Autodesk Inventor part; units mm, degrees
(part 2 of 2)
  line L135 (29.2243, -208.6026) -> (30.7211, -208.6026)
  line L136 (30.7211, -208.6026) -> (30.7211, -208.9558)
  spline S178 degree 2 poles (33.0256, -207.4318) (33.0256, -208.2519) (32.5489, -209.02) (32.0524, -209.02) knots 0 0 0 1 2 2 2
  spline S179 degree 2 poles (32.0524, -209.02) (31.5486, -209.02) (31.0768, -208.237) (31.0768, -207.4343) knots 0 0 0 1 2 2 2
  spline S180 degree 2 poles (31.0768, -207.4343) (31.0768, -206.6093) (31.5535, -205.8461) (32.0524, -205.8461) knots 0 0 0 1 2 2 2
  spline S181 degree 2 poles (32.0524, -205.8461) (32.5539, -205.8461) (33.0256, -206.6365) (33.0256, -207.4318) knots 0 0 0 1 2 2 2
  spline S182 degree 2 poles (32.502, -208.3605) (32.5613, -208.2099) (32.6107, -207.7455) (32.6107, -207.4318) knots 0 0 0 1 2 2 2
  spline S183 degree 2 poles (32.6107, -207.4318) (32.6107, -207.1181) (32.5613, -206.6562) (32.4995, -206.5006) knots 0 0 0 1 2 2 2
  spline S184 degree 2 poles (32.4995, -206.5006) (32.4378, -206.345) (32.2229, -206.1845) (32.0524, -206.1845) knots 0 0 0 1 2 2 2
  spline S185 degree 2 poles (32.0524, -206.1845) (31.882, -206.1845) (31.6622, -206.345) (31.598, -206.5056) knots 0 0 0 1 2 2 2
  spline S186 degree 2 poles (31.598, -206.5056) (31.5362, -206.6612) (31.4917, -207.1354) (31.4917, -207.4343) knots 0 0 0 1 2 2 2
  spline S187 degree 2 poles (31.4917, -207.4343) (31.4917, -207.7554) (31.5313, -208.1852) (31.5955, -208.3531) knots 0 0 0 1 2 2 2
  spline S188 degree 2 poles (31.5955, -208.3531) (31.6548, -208.5112) (31.8746, -208.6816) (32.0524, -208.6816) knots 0 0 0 1 2 2 2
  spline S189 degree 2 poles (32.0524, -208.6816) (32.2204, -208.6816) (32.4402, -208.5211) (32.502, -208.3605) knots 0 0 0 1 2 2 2
  line L137 (35.2956, -208.9558) -> (33.4159, -208.9558)
  line L138 (33.4159, -208.9558) -> (33.4159, -208.5236)
  spline S190 degree 2 poles (33.4159, -208.5236) (33.6184, -208.3334) (33.9791, -207.9802) (34.152, -207.79) knots 0 0 0 1 2 2 2
  spline S191 degree 2 poles (34.152, -207.79) (34.5002, -207.4071) (34.7546, -206.9477) (34.7546, -206.7032) knots 0 0 0 1 2 2 2
  spline S192 degree 2 poles (34.7546, -206.7032) (34.7546, -206.5747) (34.6756, -206.3821) (34.604, -206.3203) knots 0 0 0 1 2 2 2
  spline S193 degree 2 poles (34.604, -206.3203) (34.5323, -206.2586) (34.3446, -206.1968) (34.231, -206.1968) knots 0 0 0 1 2 2 2
  spline S194 degree 2 poles (34.231, -206.1968) (34.1223, -206.1968) (33.9, -206.2512) (33.7987, -206.2931) knots 0 0 0 1 2 2 2
  spline S195 degree 2 poles (33.7987, -206.2931) (33.7123, -206.3277) (33.5517, -206.4265) (33.5023, -206.4611) knots 0 0 0 1 2 2 2
  line L139 (33.5023, -206.4611) -> (33.4801, -206.4611)
  line L140 (33.4801, -206.4611) -> (33.4801, -206.0264)
  spline S196 degree 2 poles (33.4801, -206.0264) (33.6061, -205.9646) (34.0581, -205.8436) (34.2606, -205.8436) knots 0 0 0 1 2 2 2
  spline S197 degree 2 poles (34.2606, -205.8436) (34.6879, -205.8436) (35.1696, -206.2956) (35.1696, -206.6809) knots 0 0 0 1 2 2 2
  spline S198 degree 2 poles (35.1696, -206.6809) (35.1696, -206.8612) (35.0856, -207.1626) (35.0115, -207.291) knots 0 0 0 1 2 2 2
  spline S199 degree 2 poles (35.0115, -207.291) (34.9374, -207.4244) (34.7225, -207.6862) (34.604, -207.8122) knots 0 0 0 1 2 2 2
  spline S200 degree 2 poles (34.604, -207.8122) (34.4113, -208.0222) (33.9395, -208.4717) (33.7987, -208.6026) knots 0 0 0 1 2 2 2
  line L141 (33.7987, -208.6026) -> (35.2956, -208.6026)
  line L142 (35.2956, -208.6026) -> (35.2956, -208.9558)
  spline S201 degree 2 poles (37.6297, -207.9678) (37.6297, -208.2025) (37.4741, -208.6001) (37.3432, -208.7335) knots 0 0 0 1 2 2 2
  spline S202 degree 2 poles (37.3432, -208.7335) (37.2074, -208.8743) (36.8665, -209.02) (36.6615, -209.02) knots 0 0 0 1 2 2 2
  spline S203 degree 2 poles (36.6615, -209.02) (36.4565, -209.02) (36.1181, -208.8817) (35.9896, -208.7434) knots 0 0 0 1 2 2 2
  spline S204 degree 2 poles (35.9896, -208.7434) (35.8316, -208.5779) (35.6537, -208.0222) (35.6537, -207.6171) knots 0 0 0 1 2 2 2
  spline S205 degree 2 poles (35.6537, -207.6171) (35.6537, -207.2194) (35.8167, -206.5797) (35.9872, -206.3425) knots 0 0 0 1 2 2 2
  spline S206 degree 2 poles (35.9872, -206.3425) (36.1527, -206.1104) (36.6763, -205.851) (37.0196, -205.851) knots 0 0 0 1 2 2 2
  spline S207 degree 2 poles (37.0196, -205.851) (37.1209, -205.851) (37.2988, -205.8708) (37.3654, -205.893) knots 0 0 0 1 2 2 2
  line L143 (37.3654, -205.893) -> (37.3654, -206.2857)
  line L144 (37.3654, -206.2857) -> (37.3482, -206.2857)
  spline S208 degree 2 poles (37.3482, -206.2857) (37.2913, -206.2561) (37.0839, -206.2042) (36.9653, -206.2042) knots 0 0 0 1 2 2 2
  spline S209 degree 2 poles (36.9653, -206.2042) (36.5849, -206.2042) (36.1181, -206.718) (36.0736, -207.2219) knots 0 0 0 1 2 2 2
  spline S210 degree 2 poles (36.0736, -207.2219) (36.2194, -207.1206) (36.5256, -207.0094) (36.7084, -207.0094) knots 0 0 0 1 2 2 2
  spline S211 degree 2 poles (36.7084, -207.0094) (36.8863, -207.0094) (37.153, -207.0811) (37.2988, -207.1898) knots 0 0 0 1 2 2 2
  spline S212 degree 2 poles (37.2988, -207.1898) (37.4667, -207.3157) (37.6297, -207.706) (37.6297, -207.9678) knots 0 0 0 1 2 2 2
  spline S213 degree 2 poles (37.2148, -207.9851) (37.2148, -207.7974) (37.116, -207.543) (37.0073, -207.454) knots 0 0 0 1 2 2 2
  spline S214 degree 2 poles (37.0073, -207.454) (36.9258, -207.3898) (36.7232, -207.3478) (36.617, -207.3478) knots 0 0 0 1 2 2 2
  spline S215 degree 2 poles (36.617, -207.3478) (36.4738, -207.3478) (36.2045, -207.4343) (36.0736, -207.5158) knots 0 0 0 1 2 2 2
  spline S216 degree 2 poles (36.0736, -207.5158) (36.0712, -207.5603) (36.0662, -207.6442) (36.0662, -207.7085) knots 0 0 0 1 2 2 2
  spline S217 degree 2 poles (36.0662, -207.7085) (36.0662, -208.0246) (36.1897, -208.4124) (36.2836, -208.5137) knots 0 0 0 1 2 2 2
  spline S218 degree 2 poles (36.2836, -208.5137) (36.37, -208.61) (36.5578, -208.6866) (36.664, -208.6866) knots 0 0 0 1 2 2 2
  spline S219 degree 2 poles (36.664, -208.6866) (36.911, -208.6866) (37.2148, -208.3358) (37.2148, -207.9851) knots 0 0 0 1 2 2 2
  point P0 (0, 0)
  constraints: 2 other
emboss "Emboss1" sketch "Sketch14" operation cut depth 2.54 direction (-1, 0, 0)
sketch "Sketch16" plane through (5.08, 0, 0) normal (1, 0, 0) x (0, 0, -1)
  line L0 (-41.7074, -74.9522) -> (39.5726, -74.9522)
  line L1 (39.5726, -74.9522) -> (39.5726, -78.7622)
  line L2 (39.5726, -78.7622) -> (-41.7074, -78.7622)
  line L3 (-41.7074, -78.7622) -> (-41.7074, -74.9522)
  line L4 (22.7938, -210.0802) -> (-43.6417, -210.0802) projected
  point P0 (0, 0)
  point P1 (-43.6417, -212.6202)
  dimension "d193" = 135.128
  dimension "d195" = 3.81
  constraints: 8 end point, 2 parallel, 1 horizontal, 1 perpendicular
  measures "d193" distance between parallel lines of L4 L0
  measures "d195" distance between parallel lines of L0 L2
extrude "Extrusion13" add sketch "Sketch16" along normal blind 5.08
sketch "Sketch17" plane through (22.86, 33.2264, 20.9087) normal (0, 1, 0) x (1, 0, 0)
  line L0 (-6.858, 35.56) -> (0, 35.56) projected
  line L1 (-0.0061, 35.56) -> (0.0392, 35.56)
  line L2 (0, 64.9986) -> (0, -27.9146) projected
  line L3 (0, 35.5801) -> (0, 35.5243)
  line L4 (5, -24.7396) -> (5, 61.8236) projected
  line L5 (0, 35.56) -> (5, 35.56)
  line L6 (5, 35.56) -> (5, -0.0031)
  line L7 (5, -0.0031) -> (0, -0.0031)
  line L8 (0, -0.0031) -> (0, 35.56)
  point P0 (-22.86, 20.9087)
  point P1 (5, -23.8506)
  point P2 (5, 69.0626)
  point P3 (0.0392, 35.56)
  constraints: 12 end point, 4 point on line, 2 horizontal, 2 parallel, 1 perpendicular
extrude "Extrusion14" cut sketch "Sketch17" against normal blind 2.0066
sketch "Sketch18" plane through (0, 0, 0) normal (-1, 0, 0) x (0, 0, 1)
  arc A0 (46.2144, 33.1755) -> (48.7724, 30.6175) centre (48.0867, 32.4898) ccw projected
  circle A1 centre (48.0867, 32.4898) radius 4.5085
  arc A2 (-41.481, 33.1755) -> (-44.039, 30.6175) centre (-43.3533, 32.4898) ccw projected
  circle A3 centre (-43.3533, 32.4898) radius 4.5085
  arc A4 (-44.039, -212.018) -> (-41.481, -214.576) centre (-43.3533, -213.8902) ccw projected
  circle A5 centre (-43.3533, -213.8902) radius 4.5085
  arc A6 (46.2144, -214.576) -> (48.7724, -212.018) centre (48.0867, -213.8902) ccw projected
  circle A7 centre (48.0867, -213.8902) radius 4.5085
  point P0 (0, 0)
  dimension "d209" = 9.017
  dimension "d210" = 9.017
  dimension "d211" = 9.017
  dimension "d212" = 9.017
  constraints: 4 centre point, 4 coincident
  measures "d209" diameter of A1
  measures "d210" diameter of A3
  measures "d211" diameter of A5
  measures "d212" diameter of A7
extrude "Extrusion15" [suppressed]
sketch "Sketch19" plane through (22.86, -68.6784, -44.0899) normal (0, 0, -1) x (-1, 0, 0)
  line L0 (6.35, 0) -> (0, 0) projected
  line L1 (-5, 96.7232) -> (-5, -140.7668) projected
  line L2 (0, 0) -> (-5, 0)
  line L3 (-5, 0) -> (-5, 8.001)
  line L4 (-5, 8.001) -> (0, 8.001)
  line L5 (0, 8.001) -> (0, 0)
  point P0 (22.86, 68.6784)
  dimension "d216" = 5
  dimension "d219" = 8.001
  constraints: 8 end point, 2 parallel, 1 horizontal, 1 perpendicular, 1 point on line
  measures "d216" distance between parallel lines of L1 L5
  measures "d219" distance between parallel lines of L2 L4
extrude "Extrusion16" cut sketch "Sketch19" against normal blind 24.13
sketch "Sketch20" plane through (0, 0, 0) normal (-1, 0, 0) x (0, 0, 1)
  line L0 (-45.1249, 28.9592) -> (-41.5943, 28.9592)
  line L1 (-45.1249, 36.0204) -> (-41.5943, 36.0204)
  line L2 (-45.1249, 28.9592) -> (-47.1633, 32.4898)
  line L3 (-45.1249, 36.0204) -> (-47.1633, 32.4898)
  line L4 (-41.5943, 28.9592) -> (-39.5559, 32.4898)
  line L5 (-41.5943, 36.0204) -> (-39.5559, 32.4898)
  line L6 (49.8457, 36.0204) -> (51.8841, 32.4898)
  line L7 (49.8457, 28.9592) -> (51.8841, 32.4898)
  line L8 (46.3151, 28.9592) -> (49.8457, 28.9592)
  line L9 (46.3151, 36.0204) -> (49.8457, 36.0204)
  line L10 (46.3151, 36.0204) -> (44.2767, 32.4898)
  line L11 (46.3151, 28.9592) -> (44.2767, 32.4898)
  line L12 (-41.5943, -210.3596) -> (-39.5559, -213.8902)
  line L13 (-41.5943, -217.4208) -> (-39.5559, -213.8902)
  line L14 (-45.1249, -217.4208) -> (-41.5943, -217.4208)
  line L15 (-45.1249, -210.3596) -> (-41.5943, -210.3596)
  line L16 (-45.1249, -210.3596) -> (-47.1633, -213.8902)
  line L17 (-45.1249, -217.4208) -> (-47.1633, -213.8902)
  line L18 (49.8457, -210.3596) -> (51.8841, -213.8902)
  line L19 (49.8457, -217.4208) -> (51.8841, -213.8902)
  line L20 (46.3151, -217.4208) -> (49.8457, -217.4208)
  line L21 (46.3151, -210.3596) -> (49.8457, -210.3596)
  line L22 (46.3151, -210.3596) -> (44.2767, -213.8902)
  line L23 (46.3151, -217.4208) -> (44.2767, -213.8902)
  line L24 (-40.0449, -45.2596) -> (-36.5143, -45.2596)
  line L25 (-36.5143, -45.2596) -> (-34.4759, -48.7902)
  line L26 (-40.0449, -45.2596) -> (-42.0833, -48.7902)
  line L27 (-36.5143, -52.3208) -> (-34.4759, -48.7902)
  line L28 (-40.0449, -52.3208) -> (-42.0833, -48.7902)
  line L29 (-40.0449, -52.3208) -> (-36.5143, -52.3208)
  line L30 (41.2351, -45.2596) -> (39.1967, -48.7902)
  line L31 (41.2351, -52.3208) -> (39.1967, -48.7902)
  line L32 (41.2351, -45.2596) -> (44.7657, -45.2596)
  line L33 (41.2351, -52.3208) -> (44.7657, -52.3208)
  line L34 (44.7657, -52.3208) -> (46.8041, -48.7902)
  line L35 (44.7657, -45.2596) -> (46.8041, -48.7902)
  point P0 (0, 0)
  point P1 (-43.3596, 28.9592)
  point P2 (-43.3533, 32.4898)
  point P3 (48.0804, 28.9592)
  point P4 (-43.3596, -217.4208)
  point P5 (48.0804, -217.4208)
  point P6 (-38.2796, -52.3208)
  point P7 (-38.2733, -48.7902)
  point P8 (43.0004, -52.3208)
  point P9 (43.0067, -48.7902)
  dimension "d366" = 7.0612
  dimension "d367" = 120
  dimension "d368" = 120
  dimension "d369" = 120
  dimension "d370" = 120
  dimension "d371" = 3.5306
  dimension "d372" = 3.5306
  dimension "d373" = 3.5306
  dimension "d374" = 3.5306
  dimension "d375" = 3.5306
  dimension "d376" = 3.5306
  dimension "d377" = 0
  dimension "d378" = 7.6074
  dimension "d383" = 7.0612
  dimension "d384" = 120
  dimension "d385" = 120
  dimension "d386" = 120
  dimension "d387" = 120
  dimension "d388" = 3.5306
  dimension "d389" = 3.5306
  dimension "d390" = 3.5306
  dimension "d391" = 3.5306
  dimension "d392" = 3.5306
  dimension "d393" = 3.5306
  dimension "d394" = 0
  dimension "d395" = 7.6074
  dimension "d402" = 7.0612
  dimension "d403" = 120
  dimension "d404" = 120
  dimension "d405" = 120
  dimension "d406" = 120
  dimension "d407" = 3.5306
  dimension "d408" = 3.5306
  dimension "d409" = 3.5306
  dimension "d410" = 3.5306
  dimension "d411" = 3.5306
  dimension "d412" = 3.5306
  dimension "d413" = 0
  dimension "d414" = 7.6074
  dimension "d421" = 7.0612
  dimension "d422" = 120
  dimension "d423" = 120
  dimension "d424" = 120
  dimension "d425" = 120
  dimension "d426" = 3.5306
  dimension "d427" = 3.5306
  dimension "d428" = 3.5306
  dimension "d429" = 3.5306
  dimension "d430" = 3.5306
  dimension "d431" = 3.5306
  dimension "d432" = 0
  dimension "d433" = 7.6074
  dimension "d629" = 7.0612
  dimension "d630" = 120
  dimension "d631" = 120
  dimension "d632" = 120
  dimension "d633" = 120
  dimension "d634" = 3.5306
  dimension "d635" = 3.5306
  dimension "d636" = 3.5306
  dimension "d637" = 3.5306
  dimension "d638" = 3.5306
  dimension "d639" = 3.5306
  dimension "d640" = 0
  constraints: 72 end point, 12 horizontal, 6 midpoint
  measures "d366" distance from line of point (-43.36, 28.959) L1
  measures "d367" angle of L0 L2
  measures "d368" angle of L1 L3
  measures "d369" angle of L4 L0
  measures "d370" angle of L5 L1
  measures "d371" distance of L0.start L4.start
  measures "d372" distance of L1.start L5.start
  measures "d373" vertical distance of L1.start L3.end
  measures "d374" vertical distance of L0.start L2.end
  measures "d375" vertical distance of L5.start L5.end
  measures "d376" vertical distance of L4.start L4.end
  measures "d377" horizontal distance of L0.start L1.start
  measures "d378" distance of L4.end L2.end
  measures "d383" distance from line of point (48.08, 28.959) L9
  measures "d384" angle of L8 L11
  measures "d385" angle of L9 L10
  measures "d386" angle of L7 L8
  measures "d387" angle of L6 L9
  measures "d388" distance of L8.start L7.start
  measures "d389" distance of L9.start L6.start
  measures "d390" vertical distance of L9.start L10.end
  measures "d391" vertical distance of L8.start L11.end
  measures "d392" vertical distance of L6.start L6.end
  measures "d393" vertical distance of L7.start L7.end
  measures "d394" horizontal distance of L8.start L9.start
  measures "d395" distance of L7.end L11.end
  measures "d402" distance from line of point (-43.36, -217.421) L15
  measures "d403" angle of L14 L17
  measures "d404" angle of L15 L16
  measures "d405" angle of L13 L14
  measures "d406" angle of L12 L15
  measures "d407" distance of L14.start L13.start
  measures "d408" distance of L15.start L12.start
  measures "d409" vertical distance of L15.start L16.end
  measures "d410" vertical distance of L14.start L17.end
  measures "d411" vertical distance of L12.start L12.end
  measures "d412" vertical distance of L13.start L13.end
  measures "d413" horizontal distance of L14.start L15.start
  measures "d414" distance of L13.end L17.end
  measures "d421" distance from line of point (48.08, -217.421) L21
  measures "d422" angle of L20 L23
  measures "d423" angle of L21 L22
  measures "d424" angle of L19 L20
  measures "d425" angle of L18 L21
  measures "d426" distance of L20.start L19.start
  measures "d427" distance of L21.start L18.start
  measures "d428" vertical distance of L21.start L22.end
  measures "d429" vertical distance of L20.start L23.end
  measures "d430" vertical distance of L18.start L18.end
  measures "d431" vertical distance of L19.start L19.end
  measures "d432" horizontal distance of L20.start L21.start
  measures "d433" distance of L19.end L23.end
  measures "d629" distance from line of point (-38.28, -52.321) L24
  measures "d630" angle of L29 L28
  measures "d631" angle of L24 L26
  measures "d632" angle of L27 L29
  measures "d633" angle of L25 L24
  measures "d634" distance of L28.start L29.end
  measures "d635" distance of L26.start L24.end
  measures "d636" vertical distance of L26.start L26.end
  measures "d637" vertical distance of L28.start L28.end
  measures "d638" vertical distance of L24.end L25.end
  measures "d639" vertical distance of L29.end L27.end
  measures "d640" horizontal distance of L28.start L26.start
extrude "Extrusion18" cut sketch "Sketch20" against normal blind 4
sketch "Sketch21" plane through (5.08, 0, 0) normal (1, 0, 0) x (0, 0, -1)
  line L0 (42.0833, 28.0448) -> (42.0833, -209.4452) projected
  line L1 (-46.2035, -59.6599) -> (-46.8167, -60.8152)
  line L2 (-41.6901, -56.7111) -> (-44.8426, -58.3204)
  arc A0 (-44.8426, -58.3204) -> (-46.2035, -59.6599) centre (-43.399, -61.1483) ccw
  line L3 (-46.2187, -55.0206) -> (-46.361, -55.3921)
  arc A1 (-41.6901, -56.7111) -> (-39.9587, -53.8833) centre (-43.1337, -53.8833) ccw
  line L4 (-39.9587, -43.7605) -> (-39.9587, -53.8833)
  arc A2 (-39.9587, -43.7605) -> (-41.6901, -40.9327) centre (-43.1337, -43.7605) ccw
  line L5 (-41.6901, -40.9327) -> (-44.8426, -39.3233)
  line L6 (-46.2035, -37.9839) -> (-46.8167, -36.8286)
  arc A3 (-46.2035, -37.9839) -> (-44.8426, -39.3233) centre (-43.399, -36.4955) ccw
  line L7 (-46.8167, -209.4452) -> (-46.8167, 28.0448) projected
  line L8 (-46.8167, -36.8286) -> (-46.8167, -60.8152)
  circle A4 centre (-43.0067, -48.7902) radius 1.9939
  line L9 (35.2253, -54.5067) -> (35.2253, -44.384)
  line L10 (42.0833, -37.452) -> (42.0833, -61.4386)
  circle A5 centre (38.2733, -48.7902) radius 1.9939
  line L11 (42.0833, -41.6782) -> (42.0833, -55.9022)
  line L12 (35.2282, -53.9583) -> (35.2282, -43.6222)
  line L13 (36.9596, -40.7944) -> (40.1092, -39.1865)
  line L14 (41.4701, -37.8471) -> (42.0833, -36.6918)
  line L15 (36.9596, -56.7861) -> (40.1092, -58.394)
  line L16 (41.4701, -59.7334) -> (42.0833, -60.8887)
  arc A6 (36.9596, -40.7944) -> (35.2282, -43.6222) centre (38.4032, -43.6222) ccw
  arc A7 (40.1092, -39.1865) -> (41.4701, -37.8471) centre (38.6656, -36.3587) ccw
  arc A8 (35.2282, -53.9583) -> (36.9596, -56.7861) centre (38.4032, -53.9583) ccw
  arc A9 (41.4701, -59.7334) -> (40.1092, -58.394) centre (38.6656, -61.2218) ccw
  point P0 (0, 0)
  point P1 (-45.7342, -58.7756)
  point P2 (-43.0182, -55.9022)
  point P3 (-45.7342, -38.8682)
  point P4 (-43.0182, -41.6782)
  point P5 (41.0008, -38.7314)
  point P6 (41.0008, -58.8491)
  dimension "d568" = 14.224
  dimension "d569" = 2.0396
  dimension "d570" = 2.0396
  dimension "d571" = 145
  dimension "d572" = 145
  dimension "d574" = 117.044
  dimension "d575" = 117.044
  dimension "d576" = 3.175
  dimension "d577" = 6.858
  dimension "d578" = 6.858
  dimension "d579" = 7.112
  dimension "d593" = 6.858
  dimension "d594" = 6.858
  dimension "d595" = 3.9878
  dimension "d596" = 3.9878
  dimension "d598" = 0
  dimension "d600" = 3.1525
  dimension "d601" = 2.0396
  dimension "d602" = 2.0396
  dimension "d603" = 117.044
  dimension "d604" = 117.044
  dimension "d606" = 3.175
  dimension "d607" = 3.1496
  dimension "d608" = 3.1496
  dimension "d609" = 145
  dimension "d611" = 145
  constraints: 30 end point, 16 point on circle, 16 tangent, 10 centre point, 9 point on line, 6 equal radius, 2 coincident, 2 vertical, 1 parallel
  measures "d568" distance of point (-43.018, -55.902) point (-43.018, -41.678)
  measures "d569" vertical distance of point (-45.734, -38.868) L6.end
  measures "d570" vertical distance of point (-45.734, -58.776) L1.end
  measures "d571" angle of L1 L2
  measures "d572" angle of L6 L5
  measures "d574" angle of L4 L5
  measures "d575" angle of L2 L4
  measures "d576" radius of A2
  measures "d577" distance between parallel lines of L7 L4
  measures "d578" distance between parallel lines of L8 L4
  measures "d579" distance of point (-43.018, -41.678) point (-43.007, -48.79)
  measures "d593" distance between parallel lines of L10 L9
  measures "d594" distance between parallel lines of L0 L9
  measures "d595" diameter of A5
  measures "d596" diameter of A4
  measures "d598" distance between parallel lines of L0 L11
  measures "d600" horizontal distance of L5.start L5.end
  measures "d601" vertical distance of point (41.001, -58.849) L16.end
  measures "d602" vertical distance of point (41.001, -38.731) L14.end
  measures "d603" angle of L13 L12
  measures "d604" angle of L12 L15
  measures "d606" radius of A6
  measures "d607" horizontal distance of L15.start L15.end
  measures "d608" horizontal distance of L13.start L13.end
  measures "d609" angle of L15 L16
  measures "d611" angle of L13 L14
extrude "Extrusion19" add sketch "Sketch21" along normal blind 20.32
sketch "Sketch22" plane through (16.08, -218.9702, -13.3049) normal (0, -1, 0) x (1, 0, 0)
  circle A0 centre (2.2292, -12.1283) radius 2.032
  line L0 (-16.08, -35.1284) -> (6.78, -35.1284) projected
  circle A1 centre (8.732, -12.1283) radius 2.032
  line L1 (11.78, 58.9532) -> (11.78, -27.61) projected
  point P0 (-16.08, 13.3049)
  dimension "d445" = 4.064
  dimension "d446" = 23
  dimension "d449" = 4.064
  dimension "d450" = 3.048
  constraints: 2 centre point
  measures "d445" diameter of A0
  measures "d446" distance from line of L0 A0.centre
  measures "d449" diameter of A1
  measures "d450" distance from line of L1 A1.centre
extrude "Extrusion20" cut sketch "Sketch22" against normal blind 6.35
fillet "Fillet6" radius 0.508 11 edges at (19.685, -68.6784, -48.4333) (19.685, -60.6784, -48.4333) (16.51, -64.6784, -48.4333) (19.47, -218.9702, -3.3049) (16.08, -218.9702, -8.3049) (19.47, -218.9702, -13.3049) (19.431, 37.5698, -14.6513) (16.002, 37.5698, 3.1287) (19.431, 37.5698, 20.9087) (25.36, 33.2264, 20.9118) (25.36, -60.6774, -44.0899)
sketch "Sketch23" plane through (22.86, -214.6268, -13.3049) normal (0, -1, 0) x (1, 0, 0)
  line L0 (0, 10) -> (0, 58.9532) projected
  line L1 (5, 58.9532) -> (5, -27.61) projected
  line L2 (0, 10) -> (5, 10)
  line L3 (5, 10) -> (5, -0.0129)
  line L4 (5, -0.0129) -> (0, -0.0129)
  line L5 (0, -0.0129) -> (0, 10)
  point P0 (-22.86, 13.3049)
  constraints: 8 end point, 2 parallel, 1 horizontal, 1 perpendicular, 1 point on line
extrude "Extrusion21" cut sketch "Sketch23" against normal blind 6.35
body "Solid1"
